Autodesk Fusion 360 part; units mm, degrees
(part 2 of 5)
  spline S331 degree 3 poles (97.0571, -140.7904) (98.459, -139.7995) (100.4249, -139.3043) (102.9548, -139.3043) knots 0 0 0 0 1 1 1 1
  spline S332 degree 3 poles (102.9548, -139.3043) (104.6412, -139.3043) (106.2121, -139.5359) (107.6668, -139.9998) knots 0 0 0 0 1 1 1 1
  spline S333 degree 3 poles (107.6668, -139.9998) (109.132, -140.4636) (110.3496, -141.1172) (111.3196, -141.9607) knots 0 0 0 0 1 1 1 1
  line L126 (111.3196, -141.9607) -> (110.4338, -142.6721)
  spline S334 degree 3 poles (110.4338, -142.6721) (109.5695, -141.9657) (108.4839, -141.4176) (107.1766, -141.0276) knots 0 0 0 0 1 1 1 1
  spline S335 degree 3 poles (107.1766, -141.0276) (105.8693, -140.6375) (104.4624, -140.4427) (102.9548, -140.4427) knots 0 0 0 0 1 1 1 1
  spline S336 degree 3 poles (102.9548, -140.4427) (100.7303, -140.4427) (99.028, -140.8223) (97.8477, -141.5811) knots 0 0 0 0 1 1 1 1
  spline S337 degree 3 poles (97.8477, -141.5811) (96.6775, -142.3403) (96.0926, -143.3048) (96.0926, -144.4746) knots 0 0 0 0 1 1 1 1
  spline S338 degree 3 poles (96.0926, -144.4746) (96.0926, -145.7396) (96.5718, -146.715) (97.5314, -147.4001) knots 0 0 0 0 1 1 1 1
  spline S339 degree 3 poles (97.5314, -147.4001) (98.5009, -148.0746) (99.9402, -148.4119) (101.8478, -148.4119) knots 0 0 0 0 1 1 1 1
  line L127 (101.8478, -148.4119) -> (103.5875, -148.4119)
  spline S340 degree 3 poles (103.5875, -148.4119) (105.8324, -148.4119) (107.5507, -148.8653) (108.7419, -149.772) knots 0 0 0 0 1 1 1 1
  spline S341 degree 3 poles (108.7419, -149.772) (109.9436, -150.6678) (110.5444, -151.9063) (110.5444, -153.4876) knots 0 0 0 0 1 1 1 1
  spline S342 degree 3 poles (110.5444, -153.4876) (110.5444, -154.9633) (109.8435, -156.1968) (108.4415, -157.1878) knots 0 0 0 0 1 1 1 1
  spline S343 degree 3 poles (108.4415, -157.1878) (107.0396, -158.1682) (105.0737, -158.6585) (102.5438, -158.6585) knots 0 0 0 0 1 1 1 1
  spline S344 degree 3 poles (102.5438, -158.6585) (100.8569, -158.6585) (99.2811, -158.4263) (97.8158, -157.9625) knots 0 0 0 0 1 1 1 1
  spline S345 degree 3 poles (97.8158, -157.9625) (96.3611, -157.4987) (95.149, -156.845) (94.179, -156.0015) knots 0 0 0 0 1 1 1 1
  line L128 (94.179, -156.0015) -> (95.0648, -155.2901)
  spline S346 degree 3 poles (95.0648, -155.2901) (95.9292, -155.9966) (97.0147, -156.5446) (98.322, -156.9347) knots 0 0 0 0 1 1 1 1
  spline S347 degree 3 poles (98.322, -156.9347) (99.6288, -157.3248) (101.0362, -157.5196) (102.5438, -157.5196) knots 0 0 0 0 1 1 1 1
  spline S348 degree 3 poles (102.5438, -157.5196) (104.7678, -157.5196) (106.4651, -157.1404) (107.6354, -156.3812) knots 0 0 0 0 1 1 1 1
  spline S349 degree 3 poles (107.6354, -156.3812) (108.8157, -155.6224) (109.406, -154.6579) (109.406, -153.4876) knots 0 0 0 0 1 1 1 1
  spline S350 degree 3 poles (109.406, -153.4876) (109.406, -152.2227) (108.9213, -151.2527) (107.9513, -150.5781) knots 0 0 0 0 1 1 1 1
  spline S351 degree 3 poles (107.9513, -150.5781) (106.9923, -149.8931) (105.5584, -149.5503) (103.6503, -149.5503) knots 0 0 0 0 1 1 1 1
  line L129 (103.6503, -151.8276) -> (101.8478, -151.8276)
  spline S352 degree 3 poles (101.8478, -151.8276) (98.9174, -151.8276) (96.6565, -151.1635) (95.0648, -149.8353) knots 0 0 0 0 1 1 1 1
  spline S353 degree 3 poles (95.0648, -149.8353) (93.473, -148.4961) (92.6769, -146.7096) (92.6769, -144.4746) knots 0 0 0 0 1 1 1 1
  spline S354 degree 3 poles (92.6769, -144.4746) (92.6769, -143.4523) (92.9036, -142.4928) (93.3569, -141.597) knots 0 0 0 0 1 1 1 1
  spline S355 degree 3 poles (93.3569, -141.597) (93.8103, -140.7007) (94.4585, -139.9156) (95.3019, -139.241) knots 0 0 0 0 1 1 1 1
  spline S356 degree 3 poles (95.3019, -139.241) (96.1558, -138.556) (97.2414, -138.0179) (98.5592, -137.6283) knots 0 0 0 0 1 1 1 1
  spline S357 degree 3 poles (98.5592, -137.6283) (99.8769, -137.2278) (101.3421, -137.0275) (102.9548, -137.0275) knots 0 0 0 0 1 1 1 1
  spline S358 degree 3 poles (102.9548, -137.0275) (104.9895, -137.0275) (106.8921, -137.3384) (108.6627, -137.9601) knots 0 0 0 0 1 1 1 1
  spline S359 degree 3 poles (108.6627, -137.9601) (110.4338, -138.5714) (111.9095, -139.4308) (113.0903, -140.5373) knots 0 0 0 0 1 1 1 1
  line L130 (113.0903, -140.5373) -> (112.1731, -141.2174)
  spline S360 degree 3 poles (112.1731, -141.2174) (111.0979, -140.2479) (109.7538, -139.4991) (108.1411, -138.972) knots 0 0 0 0 1 1 1 1
  spline S361 degree 3 poles (108.1411, -138.972) (106.5284, -138.4344) (104.7997, -138.1659) (102.9548, -138.1659) knots 0 0 0 0 1 1 1 1
  spline S362 degree 3 poles (102.9548, -138.1659) (100.1086, -138.1659) (97.8736, -138.7667) (96.2505, -139.9684) knots 0 0 0 0 1 1 1 1
  spline S363 degree 3 poles (96.2505, -139.9684) (94.6268, -141.17) (93.8153, -142.6721) (93.8153, -144.4746) knots 0 0 0 0 1 1 1 1
  spline S364 degree 3 poles (93.8153, -144.4746) (93.8153, -146.3827) (94.5113, -147.8953) (95.9027, -149.0127) knots 0 0 0 0 1 1 1 1
  spline S365 degree 3 poles (95.9027, -149.0127) (97.2942, -150.1302) (99.2761, -150.6887) (101.8478, -150.6887) knots 0 0 0 0 1 1 1 1
  line L131 (101.8478, -150.6887) -> (103.5875, -150.6887)
  spline S366 degree 3 poles (103.5875, -150.6887) (106.7078, -150.6887) (108.2677, -151.6218) (108.2677, -153.4876) knots 0 0 0 0 1 1 1 1
  spline S367 degree 3 poles (108.2677, -153.4876) (108.2677, -154.3311) (107.7879, -155.0266) (106.8288, -155.5751) knots 0 0 0 0 1 1 1 1
  spline S368 degree 3 poles (106.8288, -155.5751) (105.8803, -156.1127) (104.4519, -156.3812) (102.5438, -156.3812) knots 0 0 0 0 1 1 1 1
  spline S369 degree 3 poles (102.5438, -156.3812) (101.2051, -156.3812) (99.9611, -156.2282) (98.8123, -155.9228) knots 0 0 0 0 1 1 1 1
  spline S370 degree 3 poles (98.8123, -155.9228) (97.6629, -155.6065) (96.7143, -155.1586) (95.966, -154.5787) knots 0 0 0 0 1 1 1 1
  line L132 (95.966, -154.5787) -> (96.8673, -153.8832)
  spline S371 degree 3 poles (96.8673, -153.8832) (98.185, -154.7894) (100.0772, -155.2428) (102.5438, -155.2428) knots 0 0 0 0 1 1 1 1
  spline S372 degree 3 poles (102.5438, -155.2428) (104.1251, -155.2428) (105.2844, -155.0794) (106.0222, -154.7525) knots 0 0 0 0 1 1 1 1
  spline S373 degree 3 poles (106.0222, -154.7525) (106.7601, -154.4257) (107.1293, -154.0042) (107.1293, -153.4876) knots 0 0 0 0 1 1 1 1
  spline S374 degree 3 poles (107.1293, -153.4876) (107.1293, -152.8868) (106.8707, -152.4598) (106.3545, -152.2067) knots 0 0 0 0 1 1 1 1
  spline S375 degree 3 poles (106.3545, -152.2067) (105.8379, -151.9536) (104.9367, -151.8276) (103.6503, -151.8276) knots 0 0 0 0 1 1 1 1
  line L133 (103.6503, -147.2735) -> (101.8478, -147.2735)
  spline S376 degree 3 poles (101.8478, -147.2735) (98.7699, -147.2735) (97.231, -146.3404) (97.231, -144.4746) knots 0 0 0 0 1 1 1 1
  spline S377 degree 3 poles (97.231, -144.4746) (97.231, -143.6317) (97.7052, -142.9412) (98.6538, -142.4036) knots 0 0 0 0 1 1 1 1
  spline S378 degree 3 poles (98.6538, -142.4036) (99.6134, -141.8551) (101.0467, -141.5811) (102.9548, -141.5811) knots 0 0 0 0 1 1 1 1
  spline S379 degree 3 poles (102.9548, -141.5811) (104.2935, -141.5811) (105.5375, -141.7395) (106.6863, -142.0553) knots 0 0 0 0 1 1 1 1
  spline S380 degree 3 poles (106.6863, -142.0553) (107.8357, -142.3612) (108.7843, -142.8041) (109.5326, -143.3836) knots 0 0 0 0 1 1 1 1
  line L134 (109.5326, -143.3836) -> (108.6313, -144.0796)
  spline S381 degree 3 poles (108.6313, -144.0796) (107.3136, -143.1728) (105.4214, -142.7195) (102.9548, -142.7195) knots 0 0 0 0 1 1 1 1
  spline S382 degree 3 poles (102.9548, -142.7195) (101.3735, -142.7195) (100.2142, -142.8829) (99.4764, -143.2097) knots 0 0 0 0 1 1 1 1
  spline S383 degree 3 poles (99.4764, -143.2097) (98.738, -143.5365) (98.3693, -143.9585) (98.3693, -144.4746) knots 0 0 0 0 1 1 1 1
  spline S384 degree 3 poles (98.3693, -144.4746) (98.3693, -145.0754) (98.6274, -145.5024) (99.1441, -145.7555) knots 0 0 0 0 1 1 1 1
  spline S385 degree 3 poles (99.1441, -145.7555) (99.6607, -146.0086) (100.5619, -146.1351) (101.8478, -146.1351) knots 0 0 0 0 1 1 1 1
  line L135 (101.8478, -146.1351) -> (103.6503, -146.1351)
  spline S386 degree 3 poles (103.6503, -146.1351) (106.5812, -146.1351) (108.8421, -146.8042) (110.4338, -148.1434) knots 0 0 0 0 1 1 1 1
  spline S387 degree 3 poles (110.4338, -148.1434) (112.0256, -149.4716) (112.8217, -151.2527) (112.8217, -153.4876) knots 0 0 0 0 1 1 1 1
  spline S388 degree 3 poles (112.8217, -153.4876) (112.8217, -154.5104) (112.595, -155.4695) (112.1417, -156.3652) knots 0 0 0 0 1 1 1 1
  spline S389 degree 3 poles (112.1417, -156.3652) (111.6883, -157.2615) (111.0347, -158.0521) (110.1807, -158.7372) knots 0 0 0 0 1 1 1 1
  spline S390 degree 3 poles (110.1807, -158.7372) (109.3378, -159.4117) (108.2572, -159.9493) (106.9394, -160.3504) knots 0 0 0 0 1 1 1 1
  spline S391 degree 3 poles (106.9394, -160.3504) (105.6217, -160.74) (104.1565, -160.9353) (102.5438, -160.9353) knots 0 0 0 0 1 1 1 1
  spline S392 degree 3 poles (102.5438, -160.9353) (100.5091, -160.9353) (98.6065, -160.6294) (96.8354, -160.0181) knots 0 0 0 0 1 1 1 1
  spline S393 degree 3 poles (96.8354, -160.0181) (95.0648, -159.3963) (93.5886, -158.5319) (92.4083, -157.4249) knots 0 0 0 0 1 1 1 1
  line L136 (92.4083, -157.4249) -> (93.325, -156.7449)
  spline S394 degree 3 poles (93.325, -156.7449) (94.4007, -157.7149) (95.7443, -158.4686) (97.3575, -159.0062) knots 0 0 0 0 1 1 1 1
  spline S395 degree 3 poles (97.3575, -159.0062) (98.9702, -159.5333) (100.6989, -159.7969) (102.5438, -159.7969) knots 0 0 0 0 1 1 1 1
  spline S396 degree 3 poles (102.5438, -159.7969) (105.39, -159.7969) (107.6245, -159.196) (109.2481, -157.9944) knots 0 0 0 0 1 1 1 1
  spline S397 degree 3 poles (109.2481, -157.9944) (110.8713, -156.7922) (111.6833, -155.2901) (111.6833, -153.4876) knots 0 0 0 0 1 1 1 1
  spline S398 degree 3 poles (111.6833, -153.4876) (111.6833, -151.5795) (110.9873, -150.067) (109.5959, -148.9495) knots 0 0 0 0 1 1 1 1
  spline S399 degree 3 poles (109.5959, -148.9495) (108.2044, -147.832) (106.2225, -147.2735) (103.6503, -147.2735) knots 0 0 0 0 1 1 1 1
  line L137 (135.7964, -154.6893) -> (135.7964, -155.8277)
  line L138 (135.7964, -155.8277) -> (126.9577, -155.8277)
  line L139 (126.9577, -155.8277) -> (127.6851, -154.6893)
  line L140 (127.6851, -154.6893) -> (135.7964, -154.6893)
  line L141 (135.7964, -156.9666) -> (135.7964, -158.105)
  line L142 (135.7964, -158.105) -> (125.5503, -158.105)
  line L143 (125.5503, -158.105) -> (126.2617, -156.9666)
  line L144 (126.2617, -156.9666) -> (135.7964, -156.9666)
  line L145 (135.7964, -159.2434) -> (135.7964, -160.3817)
  line L146 (135.7964, -160.3817) -> (124.2854, -160.3817)
  line L147 (124.2854, -160.3817) -> (124.9809, -159.2434)
  line L148 (124.9809, -159.2434) -> (135.7964, -159.2434)
  line L149 (115.1618, -143.3203) -> (115.1618, -142.1819)
  line L150 (115.1618, -142.1819) -> (124.0163, -142.1819)
  line L151 (124.0163, -142.1819) -> (123.3049, -143.3203)
  line L152 (123.3049, -143.3203) -> (115.1618, -143.3203)
  line L153 (115.1618, -141.0435) -> (115.1618, -139.9051)
  line L154 (115.1618, -139.9051) -> (125.3446, -139.9051)
  line L155 (125.3446, -139.9051) -> (124.6172, -141.0435)
  line L156 (124.6172, -141.0435) -> (115.1618, -141.0435)
  line L157 (115.1618, -138.7667) -> (115.1618, -137.6283)
  line L158 (115.1618, -137.6283) -> (126.6254, -137.6283)
  line L159 (126.6254, -137.6283) -> (125.8667, -138.7667)
  line L160 (125.8667, -138.7667) -> (115.1618, -138.7667)
  line L161 (123.1784, -160.3817) -> (121.7714, -160.3817)
  line L162 (121.7714, -160.3817) -> (135.9388, -137.6283)
  line L163 (135.9388, -137.6283) -> (135.9388, -139.5574)
  line L164 (135.9388, -139.5574) -> (123.1784, -160.3817)
  line L165 (120.364, -160.3817) -> (118.9725, -160.3817)
  line L166 (118.9725, -160.3817) -> (133.1718, -137.6283)
  line L167 (133.1718, -137.6283) -> (134.5474, -137.6283)
  line L168 (134.5474, -137.6283) -> (120.364, -160.3817)
  line L169 (117.5492, -160.3817) -> (116.1577, -160.3817)
  line L170 (116.1577, -160.3817) -> (130.3256, -137.6283)
  line L171 (130.3256, -137.6283) -> (131.733, -137.6283)
  line L172 (131.733, -137.6283) -> (117.5492, -160.3817)
  line L173 (114.7508, -160.3817) -> (114.7508, -158.0731)
  line L174 (114.7508, -158.0731) -> (127.5267, -137.6283)
  line L175 (127.5267, -137.6283) -> (128.9341, -137.6283)
  line L176 (128.9341, -137.6283) -> (114.7508, -160.3817)
  spline S400 degree 3 poles (13.712, -81.303) (13.712, -83.5618) (12.9948, -85.3972) (11.5606, -86.8101) knots 0 0 0 0 1 1 1 1
  spline S401 degree 3 poles (11.5606, -86.8101) (10.0406, -88.3301) (7.9428, -89.0899) (5.2669, -89.0899) knots 0 0 0 0 1 1 1 1
  spline S402 degree 3 poles (5.2669, -89.0899) (3.7362, -89.0899) (2.2859, -88.6938) (0.9159, -87.9022) knots 0 0 0 0 1 1 1 1
  spline S403 degree 3 poles (0.9159, -87.9022) (-0.1331, -87.3023) (-0.9305, -86.6123) (-1.4764, -85.8306) knots 0 0 0 0 1 1 1 1
  spline S404 degree 3 poles (-1.4764, -85.8306) (-1.5834, -85.178) (-1.637, -84.5836) (-1.637, -84.0486) knots 0 0 0 0 1 1 1 1
  spline S405 degree 3 poles (-1.637, -84.0486) (-1.637, -82.3039) (-1.1071, -80.9662) (-0.0475, -80.035) knots 0 0 0 0 1 1 1 1
  spline S406 degree 3 poles (-0.0475, -80.035) (0.8088, -79.2857) (1.8631, -78.9111) (3.1154, -78.9111) knots 0 0 0 0 1 1 1 1
  spline S407 degree 3 poles (3.1154, -78.9111) (4.0681, -78.9111) (4.9351, -79.1627) (5.7164, -79.6654) knots 0 0 0 0 1 1 1 1
  spline S408 degree 3 poles (5.7164, -79.6654) (6.5085, -80.2009) (7.0918, -80.9393) (7.4664, -81.8814) knots 0 0 0 0 1 1 1 1
  spline S409 degree 3 poles (7.4664, -81.8814) (7.8089, -81.8814) (7.9802, -81.7045) (7.9802, -81.3513) knots 0 0 0 0 1 1 1 1
  spline S410 degree 3 poles (7.9802, -81.3513) (7.9802, -81.1695) (7.9, -80.9288) (7.7394, -80.6289) knots 0 0 0 0 1 1 1 1
  spline S411 degree 3 poles (7.7394, -80.6289) (7.5895, -80.329) (7.3701, -80.0296) (7.0811, -79.7297) knots 0 0 0 0 1 1 1 1
  spline S412 degree 3 poles (7.0811, -79.7297) (6.3212, -78.9485) (5.406, -78.4667) (4.3357, -78.2849) knots 0 0 0 0 1 1 1 1
  line L177 (4.3357, -78.2849) -> (4.3357, -69.0367)
  spline S413 degree 3 poles (4.3357, -69.0367) (4.8708, -68.6406) (5.5452, -68.3088) (6.3586, -68.0413) knots 0 0 0 0 1 1 1 1
  spline S414 degree 3 poles (6.3586, -68.0413) (7.1721, -67.7738) (8.0979, -67.6402) (9.1362, -67.6402) knots 0 0 0 0 1 1 1 1
  spline S415 degree 3 poles (9.1362, -67.6402) (10.1745, -67.6402) (11.111, -67.8221) (11.9459, -68.1858) knots 0 0 0 0 1 1 1 1
  spline S416 degree 3 poles (11.9459, -68.1858) (13.1233, -68.7214) (13.712, -69.524) (13.712, -70.5941) knots 0 0 0 0 1 1 1 1
  line L178 (13.712, -70.5941) -> (13.712, -81.303)
  spline S417 degree 3 poles (23.7626, -81.6403) (23.8911, -81.6403) (24.0302, -81.587) (24.1801, -81.4798) knots 0 0 0 0 1 1 1 1
  spline S418 degree 3 poles (24.1801, -81.4798) (24.0731, -81.1266) (24.0195, -80.5756) (24.0195, -79.8263) knots 0 0 0 0 1 1 1 1
  line L179 (24.0195, -79.8263) -> (24.0195, -71.8949)
  spline S419 degree 3 poles (24.0195, -71.8949) (25.1541, -71.2099) (26.5188, -70.8671) (28.1137, -70.8671) knots 0 0 0 0 1 1 1 1
  spline S420 degree 3 poles (28.1137, -70.8671) (29.0128, -70.8671) (29.7995, -70.9902) (30.4738, -71.2363) knots 0 0 0 0 1 1 1 1
  spline S421 degree 3 poles (30.4738, -71.2363) (31.1588, -71.4719) (31.6833, -71.7878) (32.0472, -72.1839) knots 0 0 0 0 1 1 1 1
  line L180 (32.0472, -72.1839) -> (32.0472, -80.5487)
  spline S422 degree 3 poles (32.0472, -80.5487) (32.0472, -82.1434) (32.4326, -83.1817) (33.2032, -83.6635) knots 0 0 0 0 1 1 1 1
  spline S423 degree 3 poles (33.2032, -83.6635) (33.2139, -83.7168) (33.2193, -83.8184) (33.2193, -83.9684) knots 0 0 0 0 1 1 1 1
  line L181 (33.2193, -83.9684) -> (33.2193, -84.2573)
  spline S424 degree 3 poles (33.2193, -84.2573) (33.2193, -85.8202) (32.8072, -87.0029) (31.983, -87.8055) knots 0 0 0 0 1 1 1 1
  spline S425 degree 3 poles (31.983, -87.8055) (31.2337, -88.5548) (30.2009, -88.9295) (28.8843, -88.9295) knots 0 0 0 0 1 1 1 1
  spline S426 degree 3 poles (28.8843, -88.9295) (28.0601, -88.9295) (27.3109, -88.7421) (26.6366, -88.3675) knots 0 0 0 0 1 1 1 1
  spline S427 degree 3 poles (26.6366, -88.3675) (25.9729, -87.9928) (25.4752, -87.4468) (25.1434, -86.7299) knots 0 0 0 0 1 1 1 1
  spline S428 degree 3 poles (25.1434, -86.7299) (24.7795, -86.7299) (24.5975, -86.9068) (24.5975, -87.26) knots 0 0 0 0 1 1 1 1
  spline S429 degree 3 poles (24.5975, -87.26) (24.5975, -87.5061) (24.7206, -87.7522) (24.9668, -87.9983) knots 0 0 0 0 1 1 1 1
  spline S430 degree 3 poles (24.9668, -87.9983) (24.6243, -88.2768) (24.2122, -88.5015) (23.7306, -88.6724) knots 0 0 0 0 1 1 1 1
  spline S431 degree 3 poles (23.7306, -88.6724) (23.2489, -88.8438) (22.5371, -88.9295) (21.5952, -88.9295) knots 0 0 0 0 1 1 1 1
  spline S432 degree 3 poles (21.5952, -88.9295) (20.664, -88.9295) (19.7542, -88.7367) (18.8658, -88.3516) knots 0 0 0 0 1 1 1 1
  spline S433 degree 3 poles (18.8658, -88.3516) (17.7633, -87.8807) (16.9177, -87.1578) (16.329, -86.1839) knots 0 0 0 0 1 1 1 1
  spline S434 degree 3 poles (16.329, -86.1839) (15.6119, -85.028) (15.2533, -83.5618) (15.2533, -81.7847) knots 0 0 0 0 1 1 1 1
  line L182 (15.2533, -81.7847) -> (15.2533, -77.7548)
  spline S435 degree 3 poles (15.2533, -77.7548) (14.7074, -76.8022) (14.4345, -75.7535) (14.4345, -74.6081) knots 0 0 0 0 1 1 1 1
  spline S436 degree 3 poles (14.4345, -74.6081) (14.4345, -74.0192) (14.5094, -73.4094) (14.6592, -72.7777) knots 0 0 0 0 1 1 1 1
  spline S437 degree 3 poles (14.6592, -72.7777) (14.8091, -72.1465) (15.0499, -71.5845) (15.3817, -71.0918) knots 0 0 0 0 1 1 1 1
  line L183 (15.3817, -71.0918) -> (18.9139, -71.0918)
  spline S438 degree 3 poles (18.9139, -71.0918) (20.2411, -71.0918) (21.2794, -71.4077) (22.0286, -72.0394) knots 0 0 0 0 1 1 1 1
  spline S439 degree 3 poles (22.0286, -72.0394) (22.7886, -72.6601) (23.1686, -73.6072) (23.1686, -74.8811) knots 0 0 0 0 1 1 1 1
  line L184 (23.1686, -74.8811) -> (23.1686, -80.0829)
  spline S440 degree 3 poles (23.1686, -80.0829) (23.1686, -81.1211) (23.3666, -81.6403) (23.7626, -81.6403) knots 0 0 0 0 1 1 1 1
  spline S441 degree 3 poles (50.7197, -80.6932) (50.7197, -81.4639) (50.8054, -82.0847) (50.9763, -82.5555) knots 0 0 0 0 1 1 1 1
  spline S442 degree 3 poles (50.9763, -82.5555) (51.1477, -83.0262) (51.4476, -83.3959) (51.8755, -83.6635) knots 0 0 0 0 1 1 1 1
  spline S443 degree 3 poles (51.8755, -83.6635) (51.8865, -83.7168) (51.8915, -83.8184) (51.8915, -83.9684) knots 0 0 0 0 1 1 1 1
  line L185 (51.8915, -83.9684) -> (51.8915, -84.2573)
  spline S444 degree 3 poles (51.8915, -84.2573) (51.8915, -85.7345) (51.4635, -86.8853) (50.6071, -87.7094) knots 0 0 0 0 1 1 1 1
  spline S445 degree 3 poles (50.6071, -87.7094) (49.7617, -88.5229) (48.6646, -88.9295) (47.3159, -88.9295) knots 0 0 0 0 1 1 1 1
  spline S446 degree 3 poles (47.3159, -88.9295) (45.9779, -88.9295) (44.8915, -88.5493) (44.0566, -87.7896) knots 0 0 0 0 1 1 1 1
  spline S447 degree 3 poles (44.0566, -87.7896) (43.0826, -86.9227) (42.5956, -85.6059) (42.5956, -83.8398) knots 0 0 0 0 1 1 1 1
  spline S448 degree 3 poles (42.5956, -83.8398) (42.5956, -83.0905) (42.6277, -82.4324) (42.6919, -81.8649) knots 0 0 0 0 1 1 1 1
  spline S449 degree 3 poles (42.6919, -81.8649) (42.7668, -81.287) (42.815, -80.875) (42.8364, -80.6289) knots 0 0 0 0 1 1 1 1
  spline S450 degree 3 poles (42.8364, -80.6289) (42.8685, -80.3828) (42.9007, -80.1526) (42.9328, -79.9384) knots 0 0 0 0 1 1 1 1
  spline S451 degree 3 poles (42.9328, -79.9384) (42.9649, -79.7247) (42.9809, -79.4088) (42.9809, -78.9913) knots 0 0 0 0 1 1 1 1
  spline S452 degree 3 poles (42.9809, -78.9913) (42.9809, -78.5738) (42.922, -78.2739) (42.8043, -78.092) knots 0 0 0 0 1 1 1 1
  spline S453 degree 3 poles (42.8043, -78.092) (42.6973, -77.9102) (42.5421, -77.819) (42.3387, -77.819) knots 0 0 0 0 1 1 1 1
  spline S454 degree 3 poles (42.3387, -77.819) (42.146, -77.819) (41.9748, -77.8619) (41.8249, -77.9476) knots 0 0 0 0 1 1 1 1
  line L186 (41.8249, -77.9476) -> (42.0336, -80.5646)
  spline S455 degree 3 poles (42.0336, -80.5646) (41.841, -81.6457) (41.7447, -82.7911) (41.7447, -84.0007) knots 0 0 0 0 1 1 1 1
  spline S456 degree 3 poles (41.7447, -84.0007) (41.7447, -85.2099) (42.0176, -86.3124) (42.5635, -87.3078) knots 0 0 0 0 1 1 1 1
  spline S457 degree 3 poles (42.5635, -87.3078) (41.5145, -88.3889) (40.0428, -88.9295) (38.1483, -88.9295) knots 0 0 0 0 1 1 1 1
  spline S458 degree 3 poles (38.1483, -88.9295) (37.0672, -88.9295) (36.1306, -88.646) (35.3386, -88.0785) knots 0 0 0 0 1 1 1 1
  spline S459 degree 3 poles (35.3386, -88.0785) (34.4181, -87.4364) (33.9578, -86.5854) (33.9578, -85.5257) knots 0 0 0 0 1 1 1 1
  line L187 (33.9578, -85.5257) -> (33.9578, -66.7893)
  spline S460 degree 3 poles (33.9578, -66.7893) (34.4716, -66.4894) (35.087, -66.2433) (35.8042, -66.0505) knots 0 0 0 0 1 1 1 1
  spline S461 degree 3 poles (35.8042, -66.0505) (36.532, -65.8582) (37.2652, -65.7615) (38.0038, -65.7615) knots 0 0 0 0 1 1 1 1
  spline S462 degree 3 poles (38.0038, -65.7615) (39.2347, -65.7615) (40.2515, -66.0027) (41.0543, -66.4839) knots 0 0 0 0 1 1 1 1
  spline S463 degree 3 poles (41.0543, -66.4839) (41.9641, -67.0514) (42.419, -67.8649) (42.419, -68.9246) knots 0 0 0 0 1 1 1 1
  line L188 (42.419, -68.9246) -> (42.419, -70.4496)
  spline S464 degree 3 poles (42.419, -70.4496) (41.4878, -70.5034) (40.594, -70.771) (39.7377, -71.2527) knots 0 0 0 0 1 1 1 1
  spline S465 degree 3 poles (39.7377, -71.2527) (38.9992, -71.6807) (38.6299, -72.0713) (38.6299, -72.4245) knots 0 0 0 0 1 1 1 1
  spline S466 degree 3 poles (38.6299, -72.4245) (38.6299, -72.5426) (38.6727, -72.6492) (38.7584, -72.7458) knots 0 0 0 0 1 1 1 1
  spline S467 degree 3 poles (38.7584, -72.7458) (38.844, -72.8315) (38.9457, -72.8848) (39.0634, -72.9063) knots 0 0 0 0 1 1 1 1
  spline S468 degree 3 poles (39.0634, -72.9063) (39.513, -72.3816) (40.1445, -71.9427) (40.958, -71.5895) knots 0 0 0 0 1 1 1 1
  spline S469 degree 3 poles (40.958, -71.5895) (41.7821, -71.2363) (42.7561, -71.0599) (43.88, -71.0599) knots 0 0 0 0 1 1 1 1
  spline S470 degree 3 poles (43.88, -71.0599) (45.0039, -71.0599) (46.0154, -71.2313) (46.9145, -71.5736) knots 0 0 0 0 1 1 1 1
  spline S471 degree 3 poles (46.9145, -71.5736) (48.0488, -72.002) (48.9426, -72.6547) (49.5958, -73.5325) knots 0 0 0 0 1 1 1 1
  spline S472 degree 3 poles (49.5958, -73.5325) (50.377, -74.6026) (50.7675, -75.9463) (50.7675, -77.5625) knots 0 0 0 0 1 1 1 1
  line L189 (50.7675, -77.5625) -> (50.7197, -80.6932)
  spline S473 degree 3 poles (68.6695, -80.6932) (68.6695, -81.4639) (68.7552, -82.0847) (68.9265, -82.5555) knots 0 0 0 0 1 1 1 1
  spline S474 degree 3 poles (68.9265, -82.5555) (69.0974, -83.0262) (69.3973, -83.3959) (69.8253, -83.6635) knots 0 0 0 0 1 1 1 1
  spline S475 degree 3 poles (69.8253, -83.6635) (69.8363, -83.7168) (69.8417, -83.8184) (69.8417, -83.9684) knots 0 0 0 0 1 1 1 1
  line L190 (69.8417, -83.9684) -> (69.8417, -84.2573)
  spline S476 degree 3 poles (69.8417, -84.2573) (69.8417, -85.7773) (69.3814, -86.9601) (68.4607, -87.8055) knots 0 0 0 0 1 1 1 1
  spline S477 degree 3 poles (68.4607, -87.8055) (67.6472, -88.5548) (66.6413, -88.9295) (65.4426, -88.9295) knots 0 0 0 0 1 1 1 1
  spline S478 degree 3 poles (65.4426, -88.9295) (64.629, -88.9295) (63.8852, -88.7367) (63.2107, -88.3516) knots 0 0 0 0 1 1 1 1
  spline S479 degree 3 poles (63.2107, -88.3516) (62.5366, -87.9659) (62.0548, -87.4094) (61.7659, -86.6816) knots 0 0 0 0 1 1 1 1
  spline S480 degree 3 poles (61.7659, -86.6816) (61.4017, -86.6816) (61.2198, -86.8584) (61.2198, -87.2117) knots 0 0 0 0 1 1 1 1
  spline S481 degree 3 poles (61.2198, -87.2117) (61.2198, -87.5111) (61.4072, -87.8484) (61.7818, -88.223) knots 0 0 0 0 1 1 1 1
  spline S482 degree 3 poles (61.7818, -88.223) (61.0858, -88.6938) (60.0371, -88.9295) (58.6352, -88.9295) knots 0 0 0 0 1 1 1 1
  spline S483 degree 3 poles (58.6352, -88.9295) (56.6548, -88.9295) (55.0705, -88.3944) (53.8823, -87.3238) knots 0 0 0 0 1 1 1 1
  spline S484 degree 3 poles (53.8823, -87.3238) (52.7051, -86.2431) (52.1167, -84.7391) (52.1167, -82.8125) knots 0 0 0 0 1 1 1 1
  spline S485 degree 3 poles (52.1167, -82.8125) (52.1167, -80.875) (52.7424, -79.3764) (53.9949, -78.3167) knots 0 0 0 0 1 1 1 1
  spline S486 degree 3 poles (53.9949, -78.3167) (55.1403, -77.3642) (56.6224, -76.8879) (58.4424, -76.8879) knots 0 0 0 0 1 1 1 1
  spline S487 degree 3 poles (58.4424, -76.8879) (59.0631, -76.8879) (59.6625, -76.9307) (60.2404, -77.0164) knots 0 0 0 0 1 1 1 1
  spline S488 degree 3 poles (60.2404, -77.0164) (60.626, -77.0912) (60.8347, -77.134) (60.8666, -77.145) knots 0 0 0 0 1 1 1 1
  spline S489 degree 3 poles (60.8666, -77.145) (60.8985, -77.0379) (60.9149, -76.9467) (60.9149, -76.8719) knots 0 0 0 0 1 1 1 1
  spline S490 degree 3 poles (60.9149, -76.8719) (60.9149, -76.5935) (60.6793, -76.4061) (60.2085, -76.31) knots 0 0 0 0 1 1 1 1
  spline S491 degree 3 poles (60.2085, -76.31) (59.7372, -76.2138) (59.1219, -76.1655) (58.3621, -76.1655) knots 0 0 0 0 1 1 1 1
  spline S492 degree 3 poles (58.3621, -76.1655) (56.746, -76.1655) (55.365, -76.4918) (54.2196, -77.145) knots 0 0 0 0 1 1 1 1
  spline S493 degree 3 poles (54.2196, -77.145) (53.695, -76.2567) (53.4329, -75.1327) (53.4329, -73.7731) knots 0 0 0 0 1 1 1 1
  spline S494 degree 3 poles (53.4329, -73.7731) (53.4329, -73.0024) (53.5291, -72.43) (53.7219, -72.0553) knots 0 0 0 0 1 1 1 1
  spline S495 degree 3 poles (53.7219, -72.0553) (54.4926, -71.7021) (55.4721, -71.3917) (56.6603, -71.1242) knots 0 0 0 0 1 1 1 1
  spline S496 degree 3 poles (56.6603, -71.1242) (57.848, -70.8457) (59.1005, -70.7067) (60.4172, -70.7067) knots 0 0 0 0 1 1 1 1
  spline S497 degree 3 poles (60.4172, -70.7067) (63.1359, -70.7067) (65.191, -71.3006) (66.5825, -72.4888) knots 0 0 0 0 1 1 1 1
  spline S498 degree 3 poles (66.5825, -72.4888) (67.974, -73.677) (68.6695, -75.3629) (68.6695, -77.546) knots 0 0 0 0 1 1 1 1
  line L191 (68.6695, -77.546) -> (68.6695, -80.6932)
  spline S499 degree 3 poles (60.337, -81.4798) (59.8871, -81.4798) (59.6625, -81.6831) (59.6625, -82.0901) knots 0 0 0 0 1 1 1 1
  spline S500 degree 3 poles (59.6625, -82.0901) (59.6625, -82.4752) (59.9245, -82.668) (60.4491, -82.668) knots 0 0 0 0 1 1 1 1
  spline S501 degree 3 poles (60.4491, -82.668) (60.8133, -82.668) (61.0808, -82.5824) (61.2517, -82.411) knots 0 0 0 0 1 1 1 1
  spline S502 degree 3 poles (61.2517, -82.411) (61.4231, -82.2291) (61.5088, -81.9187) (61.5088, -81.4798) knots 0 0 0 0 1 1 1 1
  spline S503 degree 2 poles (61.5088, -81.4798) (61.1182, -81.4798) (60.337, -81.4798) knots 0 0 0 1 1 1
  spline S504 degree 3 poles (79.1053, -76.0529) (78.8273, -76.1386) (78.6878, -76.3045) (78.6878, -76.5506) knots 0 0 0 0 1 1 1 1
  line L192 (78.6878, -76.5506) -> (78.6878, -76.6313)
  spline S505 degree 3 poles (78.6878, -76.6313) (78.6878, -76.6846) (78.6933, -76.7165) (78.7043, -76.7275) knots 0 0 0 0 1 1 1 1
  spline S506 degree 3 poles (78.7043, -76.7275) (78.8219, -76.7165) (78.9773, -76.7115) (79.1696, -76.7115) knots 0 0 0 0 1 1 1 1
  line L193 (79.1696, -76.7115) -> (79.5552, -76.7115)
  spline S507 degree 3 poles (79.5552, -76.7115) (80.7753, -76.7115) (81.9152, -76.8989) (82.9749, -77.2735) knots 0 0 0 0 1 1 1 1
  spline S508 degree 3 poles (82.9749, -77.2735) (84.045, -77.6372) (84.9174, -78.2261) (85.5919, -79.0396) knots 0 0 0 0 1 1 1 1
  spline S509 degree 3 poles (85.5919, -79.0396) (86.3412, -79.9598) (86.7159, -81.1211) (86.7159, -82.5236) knots 0 0 0 0 1 1 1 1
  spline S510 degree 3 poles (86.7159, -82.5236) (86.7159, -84.7067) (85.9611, -86.3552) (84.452, -87.4682) knots 0 0 0 0 1 1 1 1
  spline S511 degree 3 poles (84.452, -87.4682) (82.943, -88.5817) (80.9253, -89.1382) (78.3989, -89.1382) knots 0 0 0 0 1 1 1 1
  spline S512 degree 3 poles (78.3989, -89.1382) (75.873, -89.1382) (73.8926, -88.7207) (72.4588, -87.8857) knots 0 0 0 0 1 1 1 1
  spline S513 degree 3 poles (72.4588, -87.8857) (71.0349, -87.0512) (70.323, -85.8257) (70.323, -84.209) knots 0 0 0 0 1 1 1 1
  spline S514 degree 3 poles (70.323, -84.209) (70.323, -83.6097) (70.4515, -83.0641) (70.7086, -82.5714) knots 0 0 0 0 1 1 1 1
  spline S515 degree 3 poles (70.7086, -82.5714) (70.9657, -82.0687) (71.2547, -81.7155) (71.5755, -81.5117) knots 0 0 0 0 1 1 1 1
  spline S516 degree 3 poles (71.5755, -81.5117) (72.1644, -82.0044) (73.0153, -82.4324) (74.1283, -82.7966) knots 0 0 0 0 1 1 1 1
  spline S517 degree 3 poles (74.1283, -82.7966) (75.2522, -83.1498) (76.4404, -83.3262) (77.6924, -83.3262) knots 0 0 0 0 1 1 1 1
  spline S518 degree 3 poles (77.6924, -83.3262) (78.1956, -83.3262) (78.4472, -83.1872) (78.4472, -82.9087) knots 0 0 0 0 1 1 1 1
  spline S519 degree 3 poles (78.4472, -82.9087) (78.4472, -82.7801) (78.4313, -82.673) (78.3989, -82.5878) knots 0 0 0 0 1 1 1 1
  spline S520 degree 3 poles (78.3989, -82.5878) (78.3241, -82.5983) (78.233, -82.6038) (78.1264, -82.6038) knots 0 0 0 0 1 1 1 1
  line L194 (78.1264, -82.6038) -> (77.9495, -82.6038)
  spline S521 degree 3 poles (77.9495, -82.6038) (75.6802, -82.6038) (73.8662, -82.1539) (72.5066, -81.2551) knots 0 0 0 0 1 1 1 1
  spline S522 degree 3 poles (72.5066, -81.2551) (70.9657, -80.2383) (70.195, -78.804) (70.195, -76.9522) knots 0 0 0 0 1 1 1 1
  spline S523 degree 3 poles (70.195, -76.9522) (70.195, -75.1003) (70.885, -73.6017) (72.266, -72.4569) knots 0 0 0 0 1 1 1 1
  spline S524 degree 3 poles (72.266, -72.4569) (73.7965, -71.1934) (75.8999, -70.5622) (78.5757, -70.5622) knots 0 0 0 0 1 1 1 1
  spline S525 degree 3 poles (78.5757, -70.5622) (79.892, -70.5622) (81.1176, -70.7012) (82.2525, -70.9797) knots 0 0 0 0 1 1 1 1
  spline S526 degree 3 poles (82.2525, -70.9797) (83.3978, -71.2577) (84.3768, -71.6274) (85.1904, -72.0872) knots 0 0 0 0 1 1 1 1
  spline S527 degree 3 poles (85.1904, -72.0872) (85.3936, -72.5261) (85.4958, -73.1738) (85.4958, -74.0302) knots 0 0 0 0 1 1 1 1
  spline S528 degree 3 poles (85.4958, -74.0302) (85.4958, -75.336) (85.1371, -76.3369) (84.4197, -77.0324) knots 0 0 0 0 1 1 1 1
  spline S529 degree 3 poles (84.4197, -77.0324) (83.8741, -76.733) (83.205, -76.4863) (82.4129, -76.294) knots 0 0 0 0 1 1 1 1
  spline S530 degree 3 poles (82.4129, -76.294) (81.6317, -76.0908) (80.9253, -75.9886) (80.2935, -75.9886) knots 0 0 0 0 1 1 1 1
  spline S531 degree 3 poles (80.2935, -75.9886) (79.6623, -75.9886) (79.2663, -76.0101) (79.1053, -76.0529) knots 0 0 0 0 1 1 1 1
  spline S532 degree 3 poles (102.9478, -75.202) (102.9478, -75.4909) (102.905, -75.9139) (102.8193, -76.4704) knots 0 0 0 0 1 1 1 1
  spline S533 degree 3 poles (102.8193, -76.4704) (102.7336, -77.0164) (102.632, -77.4554) (102.5144, -77.7871) knots 0 0 0 0 1 1 1 1
  spline S534 degree 3 poles (102.5144, -77.7871) (101.519, -79.1572) (100.3253, -80.313) (98.9338, -81.2551) knots 0 0 0 0 1 1 1 1
  spline S535 degree 3 poles (98.9338, -81.2551) (97.5638, -81.3194) (96.5579, -81.4584) (95.9157, -81.6726) knots 0 0 0 0 1 1 1 1
  spline S536 degree 3 poles (95.9157, -81.6726) (95.284, -81.8864) (94.9681, -82.1275) (94.9681, -82.395) knots 0 0 0 0 1 1 1 1
  spline S537 degree 3 poles (94.9681, -82.395) (94.9681, -82.5664) (95.0269, -82.6945) (95.145, -82.7801) knots 0 0 0 0 1 1 1 1
  spline S538 degree 3 poles (95.145, -82.7801) (95.5944, -82.534) (96.2151, -82.3412) (97.0073, -82.2022) knots 0 0 0 0 1 1 1 1
  spline S539 degree 3 poles (97.0073, -82.2022) (97.7994, -82.0523) (98.5592, -81.9775) (99.287, -81.9775) knots 0 0 0 0 1 1 1 1
  line L195 (99.287, -81.9775) -> (102.3859, -81.9775)
  spline S540 degree 3 poles (102.3859, -81.9775) (102.6639, -82.4593) (102.889, -82.9999) (103.0599, -83.5992) knots 0 0 0 0 1 1 1 1
  spline S541 degree 3 poles (103.0599, -83.5992) (103.2313, -84.1876) (103.317, -84.7067) (103.317, -85.1566) knots 0 0 0 0 1 1 1 1
  spline S542 degree 3 poles (103.317, -85.1566) (103.317, -86.3981) (102.9797, -87.3188) (102.3057, -87.9181) knots 0 0 0 0 1 1 1 1
  spline S543 degree 3 poles (102.3057, -87.9181) (101.7706, -88.3999) (101.0372, -88.6405) (100.1061, -88.6405) knots 0 0 0 0 1 1 1 1
  line L196 (100.1061, -88.6405) -> (88.6584, -88.6405)
  spline S544 degree 3 poles (88.6584, -88.6405) (87.7058, -87.6451) (87.2295, -86.0932) (87.2295, -83.9843) knots 0 0 0 0 1 1 1 1
  spline S545 degree 3 poles (87.2295, -83.9843) (87.2295, -83.2136) (87.3685, -82.2989) (87.647, -81.2392) knots 0 0 0 0 1 1 1 1
  spline S546 degree 3 poles (87.647, -81.2392) (88.621, -80.1581) (90.0015, -78.9325) (91.7891, -77.5625) knots 0 0 0 0 1 1 1 1
  spline S547 degree 3 poles (91.7891, -77.5625) (92.1423, -77.284) (92.5384, -76.9576) (92.9773, -76.583) knots 0 0 0 0 1 1 1 1
  spline S548 degree 3 poles (92.9773, -76.583) (92.913, -76.3369) (92.7686, -76.2138) (92.5439, -76.2138) knots 0 0 0 0 1 1 1 1
  spline S549 degree 3 poles (92.5439, -76.2138) (92.501, -76.2138) (92.4263, -76.2243) (92.3192, -76.2457) knots 0 0 0 0 1 1 1 1
  spline S550 degree 3 poles (92.3192, -76.2457) (92.0088, -76.3419) (91.3611, -76.8505) (90.3762, -77.7712) knots 0 0 0 0 1 1 1 1
  line L197 (90.3762, -77.7712) -> (88.3854, -77.7712)
  spline S551 degree 3 poles (88.3854, -77.7712) (87.7541, -76.733) (87.4383, -75.6195) (87.4383, -74.4313) knots 0 0 0 0 1 1 1 1
  spline S552 degree 3 poles (87.4383, -74.4313) (87.4383, -73.6825) (87.5559, -73.0189) (87.7915, -72.4404) knots 0 0 0 0 1 1 1 1
  spline S553 degree 3 poles (87.7915, -72.4404) (88.0272, -71.8625) (88.3161, -71.4131) (88.6584, -71.0918) knots 0 0 0 0 1 1 1 1
  line L198 (88.6584, -71.0918) -> (101.9041, -71.0918)
  spline S554 degree 3 poles (101.9041, -71.0918) (102.6001, -72.1086) (102.9478, -73.4787) (102.9478, -75.202) knots 0 0 0 0 1 1 1 1
  line L199 (-1.9902, -8.2305) -> (0.3738, -8.2305)
  spline S555 degree 3 poles (0.3738, -8.2305) (1.0646, -8.2305) (1.5288, -8.101) (1.7663, -7.8419) knots 0 0 0 0 1 1 1 1
  spline S556 degree 3 poles (1.7663, -7.8419) (2.0038, -7.5829) (2.1225, -7.2157) (2.1225, -6.7409) knots 0 0 0 0 1 1 1 1
  line L200 (2.1225, -6.7409) -> (2.1225, 8.1878)
  line L201 (2.1225, 8.1878) -> (9.2468, 8.1878)
  line L202 (9.2468, 8.1878) -> (9.2468, -7.9391)
  spline S557 degree 3 poles (9.2468, -7.9391) (9.2468, -9.9468) (8.7826, -11.3607) (7.8543, -12.1813) knots 0 0 0 0 1 1 1 1
  spline S558 degree 3 poles (7.8543, -12.1813) (6.9476, -13.0018) (5.4903, -13.4118) (3.4826, -13.4118) knots 0 0 0 0 1 1 1 1
  line L203 (3.4826, -13.4118) -> (-1.9902, -13.4118)
  line L204 (-1.9902, -13.4118) -> (-1.9902, -8.2305)
  spline S559 degree 3 poles (3.2235, -10.8212) (4.2814, -10.8212) (5.0262, -10.5945) (5.458, -10.1411) knots 0 0 0 0 1 1 1 1
  spline S560 degree 3 poles (5.458, -10.1411) (5.8898, -9.6663) (6.1056, -8.9644) (6.1056, -8.0362) knots 0 0 0 0 1 1 1 1
  line L205 (6.1056, -8.0362) -> (6.1056, 5.5971)
  line L206 (6.1056, 5.5971) -> (5.2313, 5.5971)
  line L207 (5.2313, 5.5971) -> (5.2313, -8.0362)
  spline S561 degree 3 poles (5.2313, -8.0362) (5.2313, -8.7053) (5.1126, -9.213) (4.8751, -9.5582) knots 0 0 0 0 1 1 1 1
  spline S562 degree 3 poles (4.8751, -9.5582) (4.6376, -9.8821) (4.0871, -10.044) (3.2235, -10.044) knots 0 0 0 0 1 1 1 1
  line L208 (3.2235, -10.044) -> (0.6005, -10.044)
  line L209 (0.6005, -10.044) -> (0.6005, -10.8212)
  line L210 (0.6005, -10.8212) -> (3.2235, -10.8212)
  spline S563 degree 3 poles (20.254, -13.9624) (18.894, -13.9624) (17.6634, -13.7895) (16.5624, -13.4442) knots 0 0 0 0 1 1 1 1
  spline S564 degree 3 poles (16.5624, -13.4442) (15.4613, -13.099) (14.5222, -12.5808) (13.745, -11.8898) knots 0 0 0 0 1 1 1 1
  spline S565 degree 3 poles (13.745, -11.8898) (12.9678, -11.1988) (12.3634, -10.3245) (11.9316, -9.2668) knots 0 0 0 0 1 1 1 1
  spline S566 degree 3 poles (11.9316, -9.2668) (11.5214, -8.2091) (11.3163, -6.9676) (11.3163, -5.5427) knots 0 0 0 0 1 1 1 1
  line L211 (11.3163, -5.5427) -> (11.3163, 8.1878)
  line L212 (11.3163, 8.1878) -> (18.2139, 8.1878)
  line L213 (18.2139, 8.1878) -> (18.2139, -5.2513)
  spline S567 degree 3 poles (18.2139, -5.2513) (18.2139, -6.007) (18.365, -6.59) (18.6673, -7) knots 0 0 0 0 1 1 1 1
  spline S568 degree 3 poles (18.6673, -7) (18.9911, -7.3886) (19.52, -7.5829) (20.254, -7.5829) knots 0 0 0 0 1 1 1 1
  spline S569 degree 3 poles (20.254, -7.5829) (20.9881, -7.5829) (21.5062, -7.3886) (21.8084, -7) knots 0 0 0 0 1 1 1 1
  spline S570 degree 3 poles (21.8084, -7) (22.1323, -6.59) (22.2942, -6.007) (22.2942, -5.2513) knots 0 0 0 0 1 1 1 1
  line L214 (22.2942, -5.2513) -> (22.2942, 8.1878)
  line L215 (22.2942, 8.1878) -> (29.2242, 8.1878)
  line L216 (29.2242, 8.1878) -> (29.2242, -5.5427)
  spline S571 degree 3 poles (29.2242, -5.5427) (29.2242, -6.9676) (29.0083, -8.2091) (28.5765, -9.2668) knots 0 0 0 0 1 1 1 1
  spline S572 degree 3 poles (28.5765, -9.2668) (28.1664, -10.3245) (27.5618, -11.1988) (26.7631, -11.8898) knots 0 0 0 0 1 1 1 1
  spline S573 degree 3 poles (26.7631, -11.8898) (25.9859, -12.5808) (25.0468, -13.099) (23.9457, -13.4442) knots 0 0 0 0 1 1 1 1
  spline S574 degree 3 poles (23.9457, -13.4442) (22.8447, -13.7895) (21.6141, -13.9624) (20.254, -13.9624) knots 0 0 0 0 1 1 1 1
  spline S575 degree 3 poles (20.254, -10.0764) (17.0157, -10.0764) (15.3966, -8.4896) (15.3966, -5.316) knots 0 0 0 0 1 1 1 1
  line L217 (15.3966, -5.316) -> (15.3966, 5.5971)
  line L218 (15.3966, 5.5971) -> (14.5546, 5.5971)
  line L219 (14.5546, 5.5971) -> (14.5546, -5.316)
  spline S576 degree 3 poles (14.5546, -5.316) (14.5546, -7.1295) (15.0404, -8.522) (16.0118, -9.4935) knots 0 0 0 0 1 1 1 1
  spline S577 degree 3 poles (16.0118, -9.4935) (17.0049, -10.4436) (18.419, -10.9183) (20.254, -10.9183) knots 0 0 0 0 1 1 1 1
  spline S578 degree 3 poles (20.254, -10.9183) (22.0891, -10.9183) (23.5032, -10.4436) (24.4962, -9.4935) knots 0 0 0 0 1 1 1 1
  spline S579 degree 3 poles (24.4962, -9.4935) (25.4893, -8.522) (25.9859, -7.1295) (25.9859, -5.316) knots 0 0 0 0 1 1 1 1
  line L220 (25.9859, -5.316) -> (25.9859, 5.5971)
  line L221 (25.9859, 5.5971) -> (25.1115, 5.5971)
  line L222 (25.1115, 5.5971) -> (25.1115, -5.316)
  spline S580 degree 3 poles (25.1115, -5.316) (25.1115, -8.4896) (23.4924, -10.0764) (20.254, -10.0764) knots 0 0 0 0 1 1 1 1
  line L223 (31.3999, 8.1878) -> (38.2976, 8.1878)
  line L224 (38.2976, 8.1878) -> (38.2976, 0.8368)
  line L225 (38.2976, 0.8368) -> (42.1512, 0.8368)
  line L226 (42.1512, 0.8368) -> (42.1512, 8.1878)
  line L227 (42.1512, 8.1878) -> (49.0811, 8.1878)
  line L228 (49.0811, 8.1878) -> (49.0811, -13.4118)
  line L229 (49.0811, -13.4118) -> (42.1512, -13.4118)
  line L230 (42.1512, -13.4118) -> (42.1512, -5.4132)
  line L231 (42.1512, -5.4132) -> (38.2976, -5.4132)
  line L232 (38.2976, -5.4132) -> (38.2976, -13.4118)
  line L233 (38.2976, -13.4118) -> (31.3999, -13.4118)
  line L234 (31.3999, -13.4118) -> (31.3999, 8.1878)
  line L235 (35.4802, -10.8212) -> (35.4802, -2.6282)
  line L236 (35.4802, -2.6282) -> (45.0009, -2.6282)
  line L237 (45.0009, -2.6282) -> (45.0009, -10.8212)
  line L238 (45.0009, -10.8212) -> (45.8429, -10.8212)
  line L239 (45.8429, -10.8212) -> (45.8429, 5.5971)
  line L240 (45.8429, 5.5971) -> (45.0009, 5.5971)
  line L241 (45.0009, 5.5971) -> (45.0009, -1.851)
  line L242 (45.0009, -1.851) -> (35.4802, -1.851)
  line L243 (35.4802, -1.851) -> (35.4802, 5.5971)
  line L244 (35.4802, 5.5971) -> (34.6383, 5.5971)
  line L245 (34.6383, 5.5971) -> (34.6383, -10.8212)
  line L246 (34.6383, -10.8212) -> (35.4802, -10.8212)
  line L247 (57.7668, 8.1878) -> (62.9481, 8.1878)
  line L248 (62.9481, 8.1878) -> (71.1411, -13.4118)
  line L249 (71.1411, -13.4118) -> (64.3406, -13.4118)
  line L250 (64.3406, -13.4118) -> (63.6282, -11.4689)
  line L251 (63.6282, -11.4689) -> (57.0868, -11.4689)
  line L252 (57.0868, -11.4689) -> (56.3743, -13.4118)
  line L253 (56.3743, -13.4118) -> (49.5738, -13.4118)
  line L254 (49.5738, -13.4118) -> (57.7668, 8.1878)
  line L255 (61.8147, -6.7085) -> (60.3575, -2.9197)
  line L256 (60.3575, -2.9197) -> (58.9002, -6.7085)
  line L257 (58.9002, -6.7085) -> (61.8147, -6.7085)
  line L258 (54.3989, -10.8212) -> (55.0142, -9.202)
  line L259 (55.0142, -9.202) -> (65.7007, -9.202)
  line L260 (65.7007, -9.202) -> (66.316, -10.8212)
  line L261 (66.316, -10.8212) -> (67.2227, -10.8212)
  line L262 (67.2227, -10.8212) -> (60.9727, 5.5971)
  line L263 (60.9727, 5.5971) -> (59.7422, 5.5971)
  line L264 (59.7422, 5.5971) -> (53.4922, -10.8212)
  line L265 (53.4922, -10.8212) -> (54.3989, -10.8212)
  line L266 (60.3575, 4.8199) -> (65.4092, -8.4248)
  line L267 (65.4092, -8.4248) -> (55.3057, -8.4248)
  line L268 (55.3057, -8.4248) -> (60.3575, 4.8199)
  spline S581 degree 3 poles (73.7631, -10.5945) (74.0655, -10.6593) (74.3893, -10.7131) (74.7346, -10.7564) knots 0 0 0 0 1 1 1 1
  spline S582 degree 3 poles (74.7346, -10.7564) (75.037, -10.7998) (75.3499, -10.8426) (75.6737, -10.8859) knots 0 0 0 0 1 1 1 1
  spline S583 degree 3 poles (75.6737, -10.8859) (76.0195, -10.9074) (76.3647, -10.9183) (76.71, -10.9183) knots 0 0 0 0 1 1 1 1
  spline S584 degree 3 poles (76.71, -10.9183) (77.3148, -10.9183) (77.8977, -10.8536) (78.4587, -10.724) knots 0 0 0 0 1 1 1 1
  spline S585 degree 3 poles (78.4587, -10.724) (79.0416, -10.5731) (79.5597, -10.3354) (80.0131, -10.0116) knots 0 0 0 0 1 1 1 1
  spline S586 degree 3 poles (80.0131, -10.0116) (80.4664, -9.6878) (80.8226, -9.2778) (81.0817, -8.781) knots 0 0 0 0 1 1 1 1
  spline S587 degree 3 poles (81.0817, -8.781) (81.3627, -8.2629) (81.5027, -7.6367) (81.5027, -6.9028) knots 0 0 0 0 1 1 1 1
  spline S588 degree 3 poles (81.5027, -6.9028) (81.5027, -6.2766) (81.3408, -5.6832) (81.0169, -5.1217) knots 0 0 0 0 1 1 1 1
  spline S589 degree 3 poles (81.0169, -5.1217) (80.715, -4.5603) (80.3155, -4.0207) (79.8188, -3.5026) knots 0 0 0 0 1 1 1 1
  spline S590 degree 3 poles (79.8188, -3.5026) (79.344, -2.9845) (78.8258, -2.4877) (78.2644, -2.013) knots 0 0 0 0 1 1 1 1
  spline S591 degree 3 poles (78.2644, -2.013) (77.7248, -1.5382) (77.2067, -1.0629) (76.71, -0.5881) knots 0 0 0 0 1 1 1 1
  spline S592 degree 3 poles (76.71, -0.5881) (76.2352, -0.0914) (75.8356, 0.3944) (75.5118, 0.8691) knots 0 0 0 0 1 1 1 1
  spline S593 degree 3 poles (75.5118, 0.8691) (75.2099, 1.3659) (75.0584, 1.873) (75.0584, 2.3912) knots 0 0 0 0 1 1 1 1
  spline S594 degree 3 poles (75.0584, 2.3912) (75.0584, 3.1684) (75.307, 3.7622) (75.8032, 4.1722) knots 0 0 0 0 1 1 1 1
  spline S595 degree 3 poles (75.8032, 4.1722) (76.3, 4.6042) (77.0986, 4.8199) (78.1996, 4.8199) knots 0 0 0 0 1 1 1 1
  spline S596 degree 3 poles (78.1996, 4.8199) (78.3725, 4.8199) (78.5453, 4.8089) (78.7177, 4.7875) knots 0 0 0 0 1 1 1 1
  spline S597 degree 3 poles (78.7177, 4.7875) (78.912, 4.7875) (79.0959, 4.7766) (79.2682, 4.7551) knots 0 0 0 0 1 1 1 1
  spline S598 degree 3 poles (79.2682, 4.7551) (79.4411, 4.7337) (79.614, 4.7227) (79.7864, 4.7227) knots 0 0 0 0 1 1 1 1
  line L269 (79.7864, 4.7227) -> (79.7864, 5.5647)
  spline S599 degree 3 poles (79.7864, 5.5647) (79.6354, 5.5647) (79.4735, 5.5757) (79.3006, 5.5971) knots 0 0 0 0 1 1 1 1
  spline S600 degree 3 poles (79.3006, 5.5971) (79.1497, 5.6185) (78.9768, 5.6295) (78.7825, 5.6295) knots 0 0 0 0 1 1 1 1
  spline S601 degree 3 poles (78.7825, 5.6295) (78.6101, 5.6509) (78.4263, 5.6619) (78.232, 5.6619) knots 0 0 0 0 1 1 1 1
  spline S602 degree 3 poles (78.232, 5.6619) (77.0662, 5.6619) (76.1057, 5.3918) (75.3499, 4.8523) knots 0 0 0 0 1 1 1 1
  spline S603 degree 3 poles (75.3499, 4.8523) (74.5946, 4.3341) (74.2165, 3.5136) (74.2165, 2.3912) knots 0 0 0 0 1 1 1 1
  spline S604 degree 3 poles (74.2165, 2.3912) (74.2165, 1.7868) (74.3679, 1.2144) (74.6698, 0.6748) knots 0 0 0 0 1 1 1 1
  spline S605 degree 3 poles (74.6698, 0.6748) (74.9937, 0.1567) (75.3932, -0.3614) (75.868, -0.8795) knots 0 0 0 0 1 1 1 1
  spline S606 degree 3 poles (75.868, -0.8795) (76.3647, -1.3762) (76.8828, -1.862) (77.4224, -2.3368) knots 0 0 0 0 1 1 1 1
  spline S607 degree 3 poles (77.4224, -2.3368) (77.9839, -2.8116) (78.502, -3.2973) (78.9768, -3.794) knots 0 0 0 0 1 1 1 1
  spline S608 degree 3 poles (78.9768, -3.794) (79.4735, -4.2688) (79.8731, -4.7655) (80.175, -5.2837) knots 0 0 0 0 1 1 1 1
  spline S609 degree 3 poles (80.175, -5.2837) (80.4988, -5.8018) (80.6607, -6.3413) (80.6607, -6.9028) knots 0 0 0 0 1 1 1 1
  spline S610 degree 3 poles (80.6607, -6.9028) (80.6607, -7.9391) (80.3045, -8.7272) (79.5921, -9.2668) knots 0 0 0 0 1 1 1 1
  spline S611 degree 3 poles (79.5921, -9.2668) (78.9016, -9.8063) (77.9405, -10.0764) (76.71, -10.0764) knots 0 0 0 0 1 1 1 1
  spline S612 degree 3 poles (76.71, -10.0764) (75.9761, -10.0764) (75.307, -10.0226) (74.7022, -9.9145) knots 0 0 0 0 1 1 1 1
  spline S613 degree 3 poles (74.7022, -9.9145) (74.3784, -9.8711) (74.0655, -9.8173) (73.7631, -9.7525) knots 0 0 0 0 1 1 1 1
  line L270 (73.7631, -9.7525) -> (73.7631, -10.5945)
  spline S614 degree 3 poles (71.0429, -6.7085) (71.5182, -6.8595) (72.0144, -6.9785) (72.5325, -7.0647) knots 0 0 0 0 1 1 1 1
  spline S615 degree 3 poles (72.5325, -7.0647) (72.9645, -7.1728) (73.4502, -7.259) (73.9898, -7.3238) knots 0 0 0 0 1 1 1 1
  spline S616 degree 3 poles (73.9898, -7.3238) (74.5513, -7.3886) (75.1127, -7.421) (75.6737, -7.421) knots 0 0 0 0 1 1 1 1
  spline S617 degree 3 poles (75.6737, -7.421) (76.6671, -7.421) (77.1633, -7.0538) (77.1633, -6.3199) knots 0 0 0 0 1 1 1 1
  spline S618 degree 3 poles (77.1633, -6.3199) (77.1633, -6.0394) (77.0124, -5.7584) (76.71, -5.478) knots 0 0 0 0 1 1 1 1
  spline S619 degree 3 poles (76.71, -5.478) (76.4081, -5.1755) (76.0195, -4.8517) (75.5442, -4.5065) knots 0 0 0 0 1 1 1 1
  spline S620 degree 3 poles (75.5442, -4.5065) (75.0908, -4.1393) (74.5946, -3.7402) (74.0546, -3.3083) knots 0 0 0 0 1 1 1 1
  spline S621 degree 3 poles (74.0546, -3.3083) (73.5364, -2.8763) (73.0402, -2.3801) (72.5649, -1.8187) knots 0 0 0 0 1 1 1 1
  spline S622 degree 3 poles (72.5649, -1.8187) (72.1116, -1.2572) (71.7339, -0.6314) (71.4315, 0.0596) knots 0 0 0 0 1 1 1 1
  spline S623 degree 3 poles (71.4315, 0.0596) (71.1296, 0.772) (70.9781, 1.5816) (70.9781, 2.4883) knots 0 0 0 0 1 1 1 1
  spline S624 degree 3 poles (70.9781, 2.4883) (70.9781, 3.5031) (71.162, 4.3989) (71.5287, 5.1761) knots 0 0 0 0 1 1 1 1
  spline S625 degree 3 poles (71.5287, 5.1761) (71.8958, 5.9533) (72.403, 6.601) (73.0507, 7.1191) knots 0 0 0 0 1 1 1 1
  spline S626 degree 3 poles (73.0507, 7.1191) (73.6983, 7.6372) (74.4541, 8.0258) (75.3175, 8.2849) knots 0 0 0 0 1 1 1 1
  spline S627 degree 3 poles (75.3175, 8.2849) (76.2028, 8.5654) (77.1419, 8.7059) (78.1348, 8.7059) knots 0 0 0 0 1 1 1 1
  spline S628 degree 3 poles (78.1348, 8.7059) (78.653, 8.7059) (79.1711, 8.6735) (79.6892, 8.6087) knots 0 0 0 0 1 1 1 1
  spline S629 degree 3 poles (79.6892, 8.6087) (80.2074, 8.5654) (80.6717, 8.5225) (81.0817, 8.4792) knots 0 0 0 0 1 1 1 1
  spline S630 degree 3 poles (81.0817, 8.4792) (81.557, 8.4144) (82.0208, 8.3497) (82.4742, 8.2849) knots 0 0 0 0 1 1 1 1
  line L271 (82.4742, 8.2849) -> (82.4742, 2.2292)
  spline S631 degree 3 poles (82.4742, 2.2292) (82.3018, 2.2507) (82.1075, 2.2726) (81.8913, 2.294) knots 0 0 0 0 1 1 1 1
  spline S632 degree 3 poles (81.8913, 2.294) (81.7189, 2.3154) (81.5246, 2.3374) (81.3084, 2.3588) knots 0 0 0 0 1 1 1 1
  spline S633 degree 3 poles (81.3084, 2.3588) (81.0927, 2.3802) (80.866, 2.3912) (80.6283, 2.3912) knots 0 0 0 0 1 1 1 1
  spline S634 degree 3 poles (80.6283, 2.3912) (80.4988, 2.3912) (80.3369, 2.3802) (80.1426, 2.3588) knots 0 0 0 0 1 1 1 1
  spline S635 degree 3 poles (80.1426, 2.3588) (79.9483, 2.3588) (79.765, 2.3374) (79.5921, 2.294) knots 0 0 0 0 1 1 1 1
  spline S636 degree 3 poles (79.5921, 2.294) (79.4197, 2.2507) (79.2682, 2.1754) (79.1387, 2.0673) knots 0 0 0 0 1 1 1 1
  spline S637 degree 3 poles (79.1387, 2.0673) (79.0092, 1.9592) (78.9444, 1.8083) (78.9444, 1.614) knots 0 0 0 0 1 1 1 1
  spline S638 degree 3 poles (78.9444, 1.614) (78.9444, 1.4411) (79.0849, 1.2254) (79.3654, 0.9663) knots 0 0 0 0 1 1 1 1
  spline S639 degree 3 poles (79.3654, 0.9663) (79.6678, 0.7072) (80.024, 0.4048) (80.434, 0.0596) knots 0 0 0 0 1 1 1 1
  spline S640 degree 3 poles (80.434, 0.0596) (80.866, -0.2857) (81.3303, -0.6852) (81.8265, -1.1386) knots 0 0 0 0 1 1 1 1
  spline S641 degree 3 poles (81.8265, -1.1386) (82.3446, -1.592) (82.809, -2.1101) (83.219, -2.693) knots 0 0 0 0 1 1 1 1
  spline S642 degree 3 poles (83.219, -2.693) (83.6509, -3.2759) (84.0072, -3.9345) (84.2876, -4.6684) knots 0 0 0 0 1 1 1 1
  spline S643 degree 3 poles (84.2876, -4.6684) (84.5901, -5.4022) (84.741, -6.2228) (84.741, -7.1295) knots 0 0 0 0 1 1 1 1
  spline S644 degree 3 poles (84.741, -7.1295) (84.741, -8.0796) (84.5901, -8.9753) (84.2876, -9.8173) knots 0 0 0 0 1 1 1 1
  spline S645 degree 3 poles (84.2876, -9.8173) (83.9857, -10.6379) (83.5104, -11.3607) (82.8628, -11.987) knots 0 0 0 0 1 1 1 1
  spline S646 degree 3 poles (82.8628, -11.987) (82.237, -12.5913) (81.4275, -13.0666) (80.434, -13.4118) knots 0 0 0 0 1 1 1 1
  spline S647 degree 3 poles (80.434, -13.4118) (79.4411, -13.779) (78.2644, -13.9624) (76.9043, -13.9624) knots 0 0 0 0 1 1 1 1
  spline S648 degree 3 poles (76.9043, -13.9624) (76.0842, -13.9624) (75.3175, -13.919) (74.6051, -13.8328) knots 0 0 0 0 1 1 1 1
  spline S649 degree 3 poles (74.6051, -13.8328) (73.9146, -13.7681) (73.2993, -13.6819) (72.7592, -13.5738) knots 0 0 0 0 1 1 1 1
  spline S650 degree 3 poles (72.7592, -13.5738) (72.1335, -13.4656) (71.561, -13.3361) (71.0429, -13.1852) knots 0 0 0 0 1 1 1 1
  line L272 (71.0429, -13.1852) -> (71.0429, -6.7085)
  line L273 (91.9366, 2.5207) -> (85.978, 2.5207)
  line L274 (85.978, 2.5207) -> (88.1801, 8.1878)
  line L275 (88.1801, 8.1878) -> (102.0077, 8.1878)
  line L276 (102.0077, 8.1878) -> (94.4948, -7.7448)
  line L277 (94.4948, -7.7448) -> (101.5867, -7.7448)